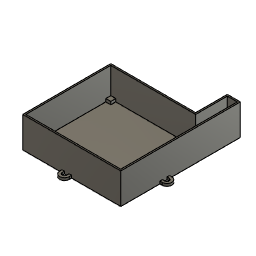
base v5 (Autodesk Fusion 360 design; units mm, degrees)
Autodesk Fusion 360 part; units mm, degrees
sketch "Sketch2" plane through (0, 0, 0) normal (0, 1, 0) x (1, 0, 0)
  line L0 (-51, 51) -> (-51, -51)
  line L1 (-51, -51) -> (63, -51)
  line L2 (63, -51) -> (63, 89)
  line L3 (63, 89) -> (51, 89)
  line L4 (51, 89) -> (51, 51)
  line L5 (51, 51) -> (-51, 51)
  dimension "d11" = 51
  dimension "d12" = 102
  dimension "d13" = 51
  dimension "d14" = 12
  dimension "d15" = 140
  dimension "d33" = 102
  constraint vertical L0
  constraint perpendicular L0 L1
  constraint perpendicular L1 L2
  constraint perpendicular L2 L3
  constraint perpendicular L3 L4
  constraint perpendicular L0 L5
  measures "d11" distance of origin L0
  measures "d12" distance of L0.start L0.end
  measures "d13" distance of origin L1
  measures "d14" distance of L2 L4
  measures "d15" distance of L1.end L2.end
  measures "d33" distance of L0.start L4.end
extrude "Extrude2" add sketch "Sketch2" along normal blind 2 makes body 1
sketch "Sketch3" plane through (0, 2, 0) normal (0, 1, 0) x (-1, 0, 0)
  line L0 (-51, -51) -> (51, -51)
  line L1 (51, -51) -> (51, 51)
  line L2 (51, 51) -> (-63, 51)
  line L3 (-63, 51) -> (-63, -89)
  line L4 (-63, -89) -> (-51, -89)
  line L5 (-51, -89) -> (-51, -51)
  line L6 (52.8, 52.8) -> (-64.8, 52.8)
  line L7 (-64.8, 52.8) -> (-64.8, -90.8)
  line L8 (-64.8, -90.8) -> (-49.2, -90.8)
  line L9 (-49.2, -90.8) -> (-49.2, -52.8)
  line L10 (-49.2, -52.8) -> (52.8, -52.8)
  line L11 (52.8, -52.8) -> (52.8, 52.8)
  dimension "d21" = 1.8
extrude "Extrude3" add sketch "Sketch3" along normal blind 35 and the other way blind 2 bodies 1
sketch "Sketch4" plane through (0, 2, 0) normal (0, 1, 0) x (-1, 0, 0)
  line L0 (-51, -51) -> (51, -51)
  line L1 (51, -51) -> (51, 51)
  line L2 (-63, -89) -> (-51, -89)
  line L3 (-51, -89) -> (-51, -51)
  line L4 (51, -51) -> (45, -51)
  line L5 (45, -51) -> (45, -45)
  line L6 (45, -45) -> (51, -45)
  line L7 (51, -45) -> (51, -51)
  line L8 (51, 51) -> (45, 51)
  line L9 (45, 51) -> (45, 45)
  line L10 (45, 45) -> (51, 45)
  line L11 (51, 45) -> (51, 51)
  line L12 (-43, -45) -> (-49, -45)
  line L13 (-49, -45) -> (-49, -51)
  line L14 (-49, -51) -> (-43, -51)
  line L15 (-43, -51) -> (-43, -45)
  line L16 (-43, 45) -> (-49, 45)
  line L17 (-49, 45) -> (-49, 51)
  line L18 (-49, 51) -> (-43, 51)
  line L19 (-43, 51) -> (-43, 45)
  dimension "d24" = 6
  dimension "d25" = 6
  dimension "d26" = 6
  dimension "d27" = 6
  dimension "d30" = 6
  dimension "d31" = 6
  dimension "d32" = 100
  dimension "d34" = 6
  dimension "d35" = 6
  dimension "d36" = 100
  constraint horizontal L4
  constraint vertical L5
  constraint horizontal L6
  constraint vertical L7
  constraint coincident L0.end L1.start
  constraint horizontal L8
  constraint vertical L9
  constraint horizontal L10
  constraint vertical L11
  constraint coincident L1.end L8.start
  constraint horizontal L12
  constraint vertical L13
  constraint horizontal L14
  constraint vertical L15
  constraint collinear L0 L14
  constraint horizontal L16
  constraint vertical L17
  constraint horizontal L18
  constraint vertical L19
  constraint collinear L10 L16
  measures "d24" distance of L5.end L6.end
  measures "d25" distance of L4.end L5.end
  measures "d26" distance of L9.end L10.end
  measures "d27" distance of L8.end L9.end
  measures "d30" distance of L12.start L14.end
  measures "d31" distance of L12.start L12.end
  measures "d32" distance of L7 L13
  measures "d34" distance of L16.start L16.end
  measures "d35" distance of L16.start L18.end
  measures "d36" distance of L11 L17
extrude "Extrude4" add sketch "Sketch4" along normal blind 3.5 bodies 1
sketch "Sketch5" plane through (0, 0, 0) normal (0, -1, 0) x (1, 0, 0)
  line L0 (-52.8, 52.8) -> (-52.8, -52.8)
  line L1 (-52.8, -52.8) -> (49.2, -52.8)
  line L2 (49.2, -52.8) -> (49.2, -90.8)
  line L3 (49.2, -90.8) -> (64.8, -90.8)
  line L4 (64.8, -90.8) -> (64.8, 52.8)
  line L5 (64.8, 52.8) -> (-52.8, 52.8)
  line L6 (-5.75, 52.8) -> (-2.75, 52.8)
  line L7 (-2.75, 52.8) -> (-2.75, 55.55)
  line L8 (-2.75, 55.55) -> (-5.75, 55.55)
  line L9 (-5.75, 55.55) -> (-5.75, 52.8)
  line L10 (5.75, 52.8) -> (2.75, 52.8)
  line L11 (2.75, 52.8) -> (2.75, 55.55)
  line L12 (2.75, 55.55) -> (5.75, 55.55)
  line L13 (5.75, 55.55) -> (5.75, 52.8)
  circle A0 centre (0, 55.55) radius 5.75
  circle A1 centre (0, 55.55) radius 2.75
  line L14 (-55.55, 5.75) -> (-55.55, 2.75)
  line L15 (-52.8, 5.75) -> (-55.55, 5.75)
  circle A2 centre (-55.55, 0) radius 2.75
  circle A3 centre (-55.55, 0) radius 5.75
  line L16 (-55.55, 2.75) -> (-52.8, 2.75)
  line L17 (-52.8, 2.75) -> (-52.8, 5.75)
  line L18 (-52.8, -5.75) -> (-55.55, -5.75)
  line L19 (-55.55, -2.75) -> (-52.8, -2.75)
  line L20 (-52.8, -2.75) -> (-52.8, -5.75)
  line L21 (-55.55, -5.75) -> (-55.55, -2.75)
  line L22 (64.8, -5.75) -> (67.55, -5.75)
  line L23 (64.8, 5.75) -> (67.55, 5.75)
  circle A4 centre (67.55, 0) radius 2.75
  line L24 (64.8, -2.75) -> (64.8, -5.75)
  line L25 (67.55, -2.75) -> (64.8, -2.75)
  line L26 (67.55, 2.75) -> (64.8, 2.75)
  line L27 (67.55, 5.75) -> (67.55, 2.75)
  line L28 (64.8, 2.75) -> (64.8, 5.75)
  circle A5 centre (67.55, 0) radius 5.75
  line L29 (67.55, -5.75) -> (67.55, -2.75)
  line L30 (2.75, -52.8) -> (5.75, -52.8)
  line L31 (-2.75, -52.8) -> (-5.75, -52.8)
  line L32 (-2.75, -55.55) -> (-2.75, -52.8)
  line L33 (-5.75, -52.8) -> (-5.75, -55.55)
  line L34 (5.75, -55.55) -> (2.75, -55.55)
  line L35 (-5.75, -55.55) -> (-2.75, -55.55)
  line L36 (2.75, -55.55) -> (2.75, -52.8)
  circle A6 centre (0, -55.55) radius 2.75
  line L37 (5.75, -52.8) -> (5.75, -55.55)
  circle A7 centre (0, -55.55) radius 5.75
  dimension "d39" = 3
  dimension "d40" = 3
  dimension "d41" = 5.5
  dimension "d42" = 5.5
  dimension "d56" = 5.5
  dimension "d57" = 3
  dimension "d62" = 2.75
  dimension "d64" = 2.75
  dimension "d66" = 5.5
  dimension "d67" = 3
  dimension "d68" = 5.5
  dimension "d69" = 3
  dimension "d70" = 2.75
  dimension "d71" = 2.75
  constraint horizontal L6
  constraint vertical L7
  constraint horizontal L8
  constraint vertical L9
  constraint coincident L5 L6.start
  constraint horizontal L10
  constraint vertical L11
  constraint horizontal L12
  constraint vertical L13
  constraint coincident L5 L10.start
  constraint concentric A0 A1
  constraint tangent L9 A0
  constraint tangent L13 A0
  constraint coincident L8 A0.centre
  constraint coincident L12 A0.centre
  constraint vertical origin A0.centre
  constraint horizontal L15
  constraint vertical L14
  constraint horizontal L16
  constraint vertical L17
  constraint horizontal L18
  constraint vertical L21
  constraint horizontal L19
  constraint vertical L20
  constraint collinear L17 L20
  constraint collinear L14 L21
  constraint concentric A2 A3
  constraint tangent A2 L16
  constraint tangent A2 L19
  constraint tangent L15 A3
  constraint tangent A3 L18
  constraint coincident L14.start A3
  constraint horizontal origin A2.centre
  constraint collinear L0 L17
  constraint horizontal L23
  constraint vertical L27
  constraint horizontal L26
  constraint vertical L28
  constraint horizontal L22
  constraint vertical L29
  constraint horizontal L25
  constraint vertical L24
  constraint collinear L24 L28
  constraint collinear L27 L29
  constraint concentric A4 A5
  constraint tangent A4 L26
  constraint tangent A4 L25
  constraint tangent L23 A5
  constraint tangent L22 A5
  constraint coincident L23.end A5
  constraint collinear L30 L31
  constraint collinear L34 L35
  constraint concentric A6 A7
  constraint tangent L36 A6
  constraint tangent L32 A6
  constraint tangent L37 A7
  constraint tangent L33 A7
  constraint coincident L34.start A7
  constraint parallel L36 L37
  constraint parallel L32 L33
  constraint perpendicular L31 L32
  constraint perpendicular L32 L35
  constraint collinear L1 L31
  constraint vertical origin A6.centre
  constraint collinear L4 L28
  constraint horizontal origin A4.centre
  measures "d39" distance of L7 L9
  measures "d40" distance of L11 L13
  measures "d41" distance of L7 L11
  measures "d42" diameter of A1
  measures "d56" distance of L16 L19
  measures "d57" distance of A2 A3
  measures "d62" distance of L6.start L8.end
  measures "d64" distance of L18.end L18.start
  measures "d66" distance of L25 L26
  measures "d67" distance of A4 A5
  measures "d68" distance of L32 L36
  measures "d69" distance of A6 A7
  measures "d70" distance of L33.end L31.end
  measures "d71" distance of L22.end L22.start
extrude "Extrude5" add sketch "Sketch5" against normal blind 3 separate body contours L0 L15 A3 L17 | L5 L6 L9 A0 | L0 L14 A3 L16 L17 | L14 A2 A3 L21 | L5 L6 L7 L8 A0 | L8 L12 A0 A1 | L0 A3 L19 L20 L21 | L0 A3 L18 L20 | L5 L10 L13 A0 | L5 L10 L11 L12 A0 | L1 L31 L33 A7 | L4 L23 L28 A5 | L1 L31 L32 L35 A7 | L34 L35 A6 A7 | L4 L26 L27 L28 A5 | A4 L27 A5 L29 | L1 L30 L34 L36 A7 | L1 L30 L37 A7 | L4 L22 L24 A5 | L4 L24 L25 A5 L29 makes body 2 at (-4.75, 0, 54.6333) makes body 3 at (-53.7167, 0, -3.75) makes body 4 at (65.7167, 0, 3.75) makes body 5 at (3.75, 0, -54.6333)
equation "d10 = 102 mm"
equation "d11 = d10 / 2"
equation "d13 = d12 / 2"
equation "d21 = ( 0.6 * 3 ) * 1 mm"
equation "d40 = d39"
equation "d42 = d41"
equation "d48 = 5.5 mm"
equation "d56 = d48"
equation "d57 = d39"
equation "d64 = d62"
equation "d66 = d48"
equation "d67 = d39"
equation "d68 = d48"
equation "d69 = d39"
equation "d70 = d62"
equation "d71 = d62"
